Autodesk Fusion 360 part; units mm, degrees
(part 4 of 6)
  spline S7 degree 5 poles (-12.9774, 23.6767) (-12.9776, 23.6654) (-12.9779, 23.6429) (-12.9782, 23.6091) (-12.9786, 23.5641) (-12.9788, 23.5079) (-12.9787, 23.4518) (-12.9784, 23.3958) (-12.9779, 23.3398) (-12.9771, 23.2839) (-12.976, 23.228) (-12.9748, 23.1723) (-12.9732, 23.1166) (-12.9714, 23.061) (-12.9694, 23.0055) (-12.9671, 22.95) (-12.9646, 22.8947) (-12.9618, 22.8394) (-12.9587, 22.7842) (-12.9554, 22.7291) (-12.9519, 22.6741) (-12.948, 22.6192) (-12.9439, 22.5643) (-12.9396, 22.5096) (-12.935, 22.4549) (-12.9301, 22.4004) (-12.9249, 22.3459) (-12.9195, 22.2915) (-12.9138, 22.2373) (-12.9078, 22.1831) (-12.9016, 22.129) (-12.895, 22.0751) (-12.8882, 22.0212) (-12.8811, 21.9675) (-12.8737, 21.9139) (-12.8661, 21.8604) (-12.8581, 21.807) (-12.8498, 21.7537) (-12.8413, 21.7006) (-12.8324, 21.6475) (-12.8233, 21.5946) (-12.8138, 21.5418) (-12.804, 21.4892) (-12.7939, 21.4367) (-12.7835, 21.3843) (-12.7728, 21.3321) (-12.7617, 21.28) (-12.7504, 21.2281) (-12.7387, 21.1763) (-12.7266, 21.1246) (-12.7143, 21.0731) (-12.7015, 21.0218) (-12.6883, 20.9707) (-12.6748, 20.9197) (-12.6609, 20.869) (-12.6466, 20.8184) (-12.632, 20.7679) (-12.617, 20.7177) (-12.6017, 20.6676) (-12.586, 20.6177) (-12.5697, 20.5681) (-12.5529, 20.5187) (-12.5355, 20.4697) (-12.5175, 20.421) (-12.4989, 20.3726) (-12.48, 20.3244) (-12.4607, 20.2763) (-12.4412, 20.2284) (-12.4213, 20.1808) (-12.4005, 20.1336) (-12.3786, 20.0871) (-12.3596, 20.0506) (-12.3444, 20.0238) (-12.3339, 20.0062) (-12.3285, 19.9974) knots -1 -1 -1 -1 -1 -1 -0.98571429 -0.97142857 -0.95714286 -0.94285714 -0.92857143 -0.91428571 -0.9 -0.88571429 -0.87142857 -0.85714286 -0.84285714 -0.82857143 -0.81428571 -0.8 -0.78571429 -0.77142857 -0.75714286 -0.74285714 -0.72857143 -0.71428571 -0.7 -0.68571429 -0.67142857 -0.65714286 -0.64285714 -0.62857143 -0.61428571 -0.6 -0.58571429 -0.57142857 -0.55714286 -0.54285714 -0.52857143 -0.51428571 -0.5 -0.48571429 -0.47142857 -0.45714286 -0.44285714 -0.42857143 -0.41428571 -0.4 -0.38571429 -0.37142857 -0.35714286 -0.34285714 -0.32857143 -0.31428571 -0.3 -0.28571429 -0.27142857 -0.25714286 -0.24285714 -0.22857143 -0.21428571 -0.2 -0.18571429 -0.17142857 -0.15714286 -0.14285714 -0.12857143 -0.11428571 -0.1 -0.08571429 -0.07142857 -0.05714286 -0.04285714 -0.02857143 -0.01428571 0 0 0 0 0 0
  line L7 (-12.3285, 19.9974) -> (-12.0674, 19.5732)
  arc A17 (-12.2216, 18.8913) -> (-12.0674, 19.5732) centre (-12.4932, 19.3111) ccw
  arc A18 (-12.2216, 18.8913) -> (-13.1932, 18.2261) centre (0, 0) ccw
  arc A19 (-13.8847, 18.3289) -> (-13.1932, 18.2261) centre (-13.4864, 18.6311) ccw
  line L8 (-13.8847, 18.3289) -> (-14.1858, 18.7257)
  spline S8 degree 5 poles (-14.1858, 18.7257) (-14.192, 18.7339) (-14.2046, 18.7501) (-14.2242, 18.774) (-14.2513, 18.8048) (-14.2867, 18.8421) (-14.3232, 18.8785) (-14.3604, 18.9144) (-14.398, 18.9499) (-14.4358, 18.9852) (-14.4739, 19.0203) (-14.5124, 19.0551) (-14.5513, 19.0895) (-14.5907, 19.1235) (-14.6306, 19.157) (-14.671, 19.1901) (-14.7118, 19.2228) (-14.753, 19.2552) (-14.7944, 19.2873) (-14.8361, 19.3192) (-14.8781, 19.3508) (-14.9204, 19.3821) (-14.963, 19.4131) (-15.006, 19.4439) (-15.0492, 19.4744) (-15.0927, 19.5045) (-15.1365, 19.5344) (-15.1806, 19.5641) (-15.2249, 19.5935) (-15.2695, 19.6226) (-15.3143, 19.6515) (-15.3593, 19.6801) (-15.4046, 19.7085) (-15.4502, 19.7367) (-15.496, 19.7646) (-15.542, 19.7923) (-15.5882, 19.8197) (-15.6347, 19.8469) (-15.6814, 19.8739) (-15.7283, 19.9006) (-15.7754, 19.9271) (-15.8227, 19.9534) (-15.8702, 19.9794) (-15.918, 20.0052) (-15.9659, 20.0308) (-16.014, 20.0562) (-16.0624, 20.0814) (-16.1109, 20.1063) (-16.1596, 20.131) (-16.2085, 20.1555) (-16.2576, 20.1798) (-16.3069, 20.2039) (-16.3564, 20.2278) (-16.406, 20.2514) (-16.4559, 20.2748) (-16.5059, 20.2981) (-16.5561, 20.3211) (-16.6064, 20.3439) (-16.6569, 20.3665) (-16.7076, 20.3889) (-16.7585, 20.411) (-16.8095, 20.433) (-16.8607, 20.4548) (-16.9121, 20.4763) (-16.9636, 20.4977) (-17.0153, 20.5189) (-17.0671, 20.5398) (-17.1191, 20.5606) (-17.1713, 20.5811) (-17.2236, 20.6014) (-17.276, 20.6216) (-17.3181, 20.6375) (-17.3497, 20.6494) (-17.3709, 20.6573) (-17.3814, 20.6612) knots 0 0 0 0 0 0 0.01428571 0.02857143 0.04285714 0.05714286 0.07142857 0.08571429 0.1 0.11428571 0.12857143 0.14285714 0.15714286 0.17142857 0.18571429 0.2 0.21428571 0.22857143 0.24285714 0.25714286 0.27142857 0.28571429 0.3 0.31428571 0.32857143 0.34285714 0.35714286 0.37142857 0.38571429 0.4 0.41428571 0.42857143 0.44285714 0.45714286 0.47142857 0.48571429 0.5 0.51428571 0.52857143 0.54285714 0.55714286 0.57142857 0.58571429 0.6 0.61428571 0.62857143 0.64285714 0.65714286 0.67142857 0.68571429 0.7 0.71428571 0.72857143 0.74285714 0.75714286 0.77142857 0.78571429 0.8 0.81428571 0.82857143 0.84285714 0.85714286 0.87142857 0.88571429 0.9 0.91428571 0.92857143 0.94285714 0.95714286 0.97142857 0.98571429 1 1 1 1 1 1
  arc A20 (-17.3814, 20.6612) -> (-18.4579, 19.7055) centre (0, 0) ccw
  spline S9 degree 5 poles (-18.4579, 19.7055) (-18.4552, 19.6946) (-18.4499, 19.6727) (-18.4418, 19.6398) (-18.431, 19.5962) (-18.4172, 19.5417) (-18.4032, 19.4874) (-18.389, 19.4331) (-18.3745, 19.3791) (-18.3598, 19.3251) (-18.345, 19.2713) (-18.3298, 19.2176) (-18.3145, 19.1641) (-18.299, 19.1106) (-18.2832, 19.0574) (-18.2672, 19.0042) (-18.251, 18.9512) (-18.2345, 18.8984) (-18.2178, 18.8457) (-18.2009, 18.7931) (-18.1838, 18.7407) (-18.1664, 18.6885) (-18.1488, 18.6364) (-18.131, 18.5844) (-18.1129, 18.5327) (-18.0946, 18.481) (-18.0761, 18.4296) (-18.0573, 18.3782) (-18.0383, 18.3271) (-18.019, 18.2761) (-17.9995, 18.2253) (-17.9798, 18.1747) (-17.9598, 18.1242) (-17.9395, 18.074) (-17.919, 18.0239) (-17.8983, 17.9739) (-17.8773, 17.9242) (-17.8561, 17.8746) (-17.8346, 17.8253) (-17.8128, 17.7761) (-17.7908, 17.7272) (-17.7685, 17.6784) (-17.7459, 17.6298) (-17.7231, 17.5815) (-17.7, 17.5334) (-17.6766, 17.4854) (-17.6529, 17.4377) (-17.629, 17.3902) (-17.6048, 17.343) (-17.5803, 17.2959) (-17.5555, 17.2492) (-17.5304, 17.2026) (-17.5049, 17.1564) (-17.4791, 17.1104) (-17.453, 17.0647) (-17.4266, 17.0192) (-17.3999, 16.974) (-17.3729, 16.9291) (-17.3456, 16.8844) (-17.318, 16.84) (-17.2899, 16.7959) (-17.2614, 16.7523) (-17.2323, 16.7092) (-17.2027, 16.6665) (-17.1727, 16.6242) (-17.1424, 16.5822) (-17.1118, 16.5405) (-17.081, 16.4989) (-17.0498, 16.4577) (-17.018, 16.4172) (-16.9851, 16.3776) (-16.9577, 16.347) (-16.9363, 16.3248) (-16.9217, 16.3104) (-16.9143, 16.3032) knots -1 -1 -1 -1 -1 -1 -0.98571429 -0.97142857 -0.95714286 -0.94285714 -0.92857143 -0.91428571 -0.9 -0.88571429 -0.87142857 -0.85714286 -0.84285714 -0.82857143 -0.81428571 -0.8 -0.78571429 -0.77142857 -0.75714286 -0.74285714 -0.72857143 -0.71428571 -0.7 -0.68571429 -0.67142857 -0.65714286 -0.64285714 -0.62857143 -0.61428571 -0.6 -0.58571429 -0.57142857 -0.55714286 -0.54285714 -0.52857143 -0.51428571 -0.5 -0.48571429 -0.47142857 -0.45714286 -0.44285714 -0.42857143 -0.41428571 -0.4 -0.38571429 -0.37142857 -0.35714286 -0.34285714 -0.32857143 -0.31428571 -0.3 -0.28571429 -0.27142857 -0.25714286 -0.24285714 -0.22857143 -0.21428571 -0.2 -0.18571429 -0.17142857 -0.15714286 -0.14285714 -0.12857143 -0.11428571 -0.1 -0.08571429 -0.07142857 -0.05714286 -0.04285714 -0.02857143 -0.01428571 0 0 0 0 0 0
  line L9 (-16.9143, 16.3032) -> (-16.5559, 15.9572)
  arc A21 (-16.5357, 15.2584) -> (-16.5559, 15.9572) centre (-16.9032, 15.5975) ccw
  arc A22 (-16.5357, 15.2584) -> (-17.3113, 14.3724) centre (0, 0) ccw
  arc A23 (-18.0067, 14.3) -> (-17.3113, 14.3724) centre (-17.696, 14.6918) ccw
  line L10 (-18.0067, 14.3) -> (-18.397, 14.6095)
  spline S10 degree 5 poles (-18.397, 14.6095) (-18.4051, 14.6159) (-18.4213, 14.6285) (-18.4462, 14.6467) (-18.4801, 14.6699) (-18.5237, 14.6972) (-18.5681, 14.7234) (-18.6131, 14.7488) (-18.6583, 14.7739) (-18.7037, 14.7987) (-18.7494, 14.8232) (-18.7953, 14.8474) (-18.8415, 14.871) (-18.8881, 14.8941) (-18.9351, 14.9166) (-18.9824, 14.9386) (-19.0301, 14.9602) (-19.078, 14.9813) (-19.1262, 15.0021) (-19.1745, 15.0226) (-19.2231, 15.0428) (-19.2718, 15.0626) (-19.3208, 15.0821) (-19.37, 15.1012) (-19.4195, 15.12) (-19.4691, 15.1384) (-19.519, 15.1564) (-19.569, 15.1742) (-19.6193, 15.1916) (-19.6697, 15.2088) (-19.7203, 15.2256) (-19.771, 15.2421) (-19.822, 15.2584) (-19.8731, 15.2743) (-19.9244, 15.29) (-19.9758, 15.3053) (-20.0274, 15.3204) (-20.0792, 15.3352) (-20.1311, 15.3497) (-20.1832, 15.3639) (-20.2354, 15.3779) (-20.2878, 15.3915) (-20.3403, 15.405) (-20.393, 15.4181) (-20.4458, 15.431) (-20.4987, 15.4436) (-20.5518, 15.4559) (-20.605, 15.468) (-20.6583, 15.4798) (-20.7118, 15.4914) (-20.7654, 15.5027) (-20.8191, 15.5138) (-20.873, 15.5246) (-20.9269, 15.5352) (-20.981, 15.5455) (-21.0352, 15.5555) (-21.0896, 15.5653) (-21.144, 15.5749) (-21.1986, 15.5842) (-21.2532, 15.5933) (-21.308, 15.6021) (-21.3629, 15.6107) (-21.4179, 15.6191) (-21.473, 15.6272) (-21.5282, 15.6351) (-21.5836, 15.6427) (-21.639, 15.6501) (-21.6945, 15.6573) (-21.7501, 15.6642) (-21.8058, 15.6709) (-21.8616, 15.6774) (-21.9064, 15.6823) (-21.94, 15.686) (-21.9624, 15.6884) (-21.9736, 15.6895) knots 0 0 0 0 0 0 0.01428571 0.02857143 0.04285714 0.05714286 0.07142857 0.08571429 0.1 0.11428571 0.12857143 0.14285714 0.15714286 0.17142857 0.18571429 0.2 0.21428571 0.22857143 0.24285714 0.25714286 0.27142857 0.28571429 0.3 0.31428571 0.32857143 0.34285714 0.35714286 0.37142857 0.38571429 0.4 0.41428571 0.42857143 0.44285714 0.45714286 0.47142857 0.48571429 0.5 0.51428571 0.52857143 0.54285714 0.55714286 0.57142857 0.58571429 0.6 0.61428571 0.62857143 0.64285714 0.65714286 0.67142857 0.68571429 0.7 0.71428571 0.72857143 0.74285714 0.75714286 0.77142857 0.78571429 0.8 0.81428571 0.82857143 0.84285714 0.85714286 0.87142857 0.88571429 0.9 0.91428571 0.92857143 0.94285714 0.95714286 0.97142857 0.98571429 1 1 1 1 1 1
  arc A24 (-21.9736, 15.6895) -> (-22.7785, 14.4962) centre (0, 0) ccw
  spline S11 degree 5 poles (-22.7785, 14.4962) (-22.7732, 14.4862) (-22.7626, 14.4663) (-22.7467, 14.4365) (-22.7253, 14.3969) (-22.6984, 14.3476) (-22.6713, 14.2984) (-22.6441, 14.2495) (-22.6166, 14.2007) (-22.589, 14.1521) (-22.5612, 14.1036) (-22.5332, 14.0554) (-22.505, 14.0073) (-22.4767, 13.9595) (-22.4482, 13.9118) (-22.4194, 13.8643) (-22.3906, 13.817) (-22.3615, 13.7699) (-22.3322, 13.723) (-22.3028, 13.6763) (-22.2731, 13.6298) (-22.2433, 13.5836) (-22.2133, 13.5375) (-22.1831, 13.4916) (-22.1527, 13.4459) (-22.1222, 13.4005) (-22.0914, 13.3552) (-22.0605, 13.3102) (-22.0293, 13.2654) (-21.998, 13.2208) (-21.9665, 13.1764) (-21.9348, 13.1323) (-21.9028, 13.0884) (-21.8707, 13.0447) (-21.8384, 13.0013) (-21.8059, 12.9581) (-21.7732, 12.9152) (-21.7403, 12.8725) (-21.7072, 12.83) (-21.6739, 12.7878) (-21.6404, 12.7458) (-21.6067, 12.7041) (-21.5728, 12.6627) (-21.5386, 12.6216) (-21.5043, 12.5807) (-21.4697, 12.5401) (-21.4349, 12.4998) (-21.3999, 12.4597) (-21.3647, 12.42) (-21.3293, 12.3805) (-21.2936, 12.3414) (-21.2577, 12.3026) (-21.2216, 12.2641) (-21.1852, 12.226) (-21.1485, 12.1882) (-21.1116, 12.1507) (-21.0745, 12.1136) (-21.0372, 12.0767) (-20.9996, 12.0402) (-20.9618, 12.0041) (-20.9237, 11.9684) (-20.8852, 11.9333) (-20.8463, 11.8987) (-20.8071, 11.8647) (-20.7675, 11.8312) (-20.7276, 11.7981) (-20.6876, 11.7653) (-20.6475, 11.7327) (-20.607, 11.7006) (-20.5661, 11.6692) (-20.5245, 11.639) (-20.4903, 11.6162) (-20.4641, 11.6) (-20.4463, 11.5897) (-20.4374, 11.5846) knots -1 -1 -1 -1 -1 -1 -0.98571429 -0.97142857 -0.95714286 -0.94285714 -0.92857143 -0.91428571 -0.9 -0.88571429 -0.87142857 -0.85714286 -0.84285714 -0.82857143 -0.81428571 -0.8 -0.78571429 -0.77142857 -0.75714286 -0.74285714 -0.72857143 -0.71428571 -0.7 -0.68571429 -0.67142857 -0.65714286 -0.64285714 -0.62857143 -0.61428571 -0.6 -0.58571429 -0.57142857 -0.55714286 -0.54285714 -0.52857143 -0.51428571 -0.5 -0.48571429 -0.47142857 -0.45714286 -0.44285714 -0.42857143 -0.41428571 -0.4 -0.38571429 -0.37142857 -0.35714286 -0.34285714 -0.32857143 -0.31428571 -0.3 -0.28571429 -0.27142857 -0.25714286 -0.24285714 -0.22857143 -0.21428571 -0.2 -0.18571429 -0.17142857 -0.15714286 -0.14285714 -0.12857143 -0.11428571 -0.1 -0.08571429 -0.07142857 -0.05714286 -0.04285714 -0.02857143 -0.01428571 0 0 0 0 0 0
  line L11 (-20.4374, 11.5846) -> (-20.0042, 11.3386)
  arc A25 (-19.8108, 10.6668) -> (-20.0042, 11.3386) centre (-20.2511, 10.9038) ccw
  arc A26 (-19.8108, 10.6668) -> (-20.3418, 9.6158) centre (0, 0) ccw
  arc A27 (-20.9972, 9.3727) -> (-20.3418, 9.6158) centre (-20.7938, 9.8294) ccw
  line L12 (-20.9972, 9.3727) -> (-21.4523, 9.5754)
  spline S12 degree 5 poles (-21.4523, 9.5754) (-21.4617, 9.5796) (-21.4806, 9.5877) (-21.5092, 9.5992) (-21.5478, 9.6132) (-21.5968, 9.6288) (-21.6463, 9.6431) (-21.6962, 9.6566) (-21.7462, 9.6696) (-21.7964, 9.6823) (-21.8467, 9.6947) (-21.8972, 9.7067) (-21.9478, 9.7181) (-21.9987, 9.7289) (-22.0498, 9.7391) (-22.1012, 9.7486) (-22.1527, 9.7576) (-22.2044, 9.7661) (-22.2562, 9.7743) (-22.3081, 9.7821) (-22.3601, 9.7896) (-22.4123, 9.7967) (-22.4646, 9.8034) (-22.517, 9.8096) (-22.5695, 9.8155) (-22.6222, 9.821) (-22.675, 9.8261) (-22.7279, 9.8308) (-22.7809, 9.8352) (-22.834, 9.8393) (-22.8872, 9.843) (-22.9405, 9.8464) (-22.9938, 9.8495) (-23.0473, 9.8522) (-23.1009, 9.8546) (-23.1545, 9.8567) (-23.2083, 9.8585) (-23.2621, 9.8599) (-23.316, 9.861) (-23.37, 9.8619) (-23.424, 9.8624) (-23.4781, 9.8626) (-23.5323, 9.8626) (-23.5866, 9.8622) (-23.641, 9.8615) (-23.6954, 9.8606) (-23.7498, 9.8593) (-23.8044, 9.8578) (-23.859, 9.856) (-23.9137, 9.8539) (-23.9684, 9.8515) (-24.0232, 9.8489) (-24.078, 9.846) (-24.1329, 9.8428) (-24.1879, 9.8393) (-24.2429, 9.8356) (-24.2979, 9.8316) (-24.3531, 9.8273) (-24.4082, 9.8227) (-24.4634, 9.8179) (-24.5187, 9.8129) (-24.574, 9.8075) (-24.6293, 9.8019) (-24.6847, 9.7961) (-24.7402, 9.79) (-24.7956, 9.7836) (-24.8512, 9.777) (-24.9067, 9.7702) (-24.9623, 9.763) (-25.0179, 9.7557) (-25.0736, 9.7481) (-25.1182, 9.7418) (-25.1516, 9.7369) (-25.1739, 9.7337) (-25.1851, 9.732) knots 0 0 0 0 0 0 0.01428571 0.02857143 0.04285714 0.05714286 0.07142857 0.08571429 0.1 0.11428571 0.12857143 0.14285714 0.15714286 0.17142857 0.18571429 0.2 0.21428571 0.22857143 0.24285714 0.25714286 0.27142857 0.28571429 0.3 0.31428571 0.32857143 0.34285714 0.35714286 0.37142857 0.38571429 0.4 0.41428571 0.42857143 0.44285714 0.45714286 0.47142857 0.48571429 0.5 0.51428571 0.52857143 0.54285714 0.55714286 0.57142857 0.58571429 0.6 0.61428571 0.62857143 0.64285714 0.65714286 0.67142857 0.68571429 0.7 0.71428571 0.72857143 0.74285714 0.75714286 0.77142857 0.78571429 0.8 0.81428571 0.82857143 0.84285714 0.85714286 0.87142857 0.88571429 0.9 0.91428571 0.92857143 0.94285714 0.95714286 0.97142857 0.98571429 1 1 1 1 1 1
  arc A28 (-25.1851, 9.732) -> (-25.6679, 8.3759) centre (0, 0) ccw
  spline S13 degree 5 poles (-25.6679, 8.3759) (-25.6603, 8.3676) (-25.6451, 8.351) (-25.6223, 8.3261) (-25.5917, 8.2931) (-25.5534, 8.252) (-25.5149, 8.2111) (-25.4763, 8.1704) (-25.4376, 8.13) (-25.3988, 8.0898) (-25.3598, 8.0498) (-25.3207, 8.01) (-25.2815, 7.9705) (-25.2421, 7.9312) (-25.2026, 7.8921) (-25.163, 7.8533) (-25.1233, 7.8146) (-25.0834, 7.7763) (-25.0434, 7.7381) (-25.0033, 7.7002) (-24.963, 7.6625) (-24.9226, 7.6251) (-24.8821, 7.5879) (-24.8414, 7.551) (-24.8006, 7.5143) (-24.7597, 7.4779) (-24.7187, 7.4417) (-24.6775, 7.4058) (-24.6362, 7.3702) (-24.5948, 7.3348) (-24.5532, 7.2996) (-24.5115, 7.2648) (-24.4697, 7.2302) (-24.4277, 7.1959) (-24.3856, 7.1619) (-24.3434, 7.1281) (-24.3011, 7.0946) (-24.2586, 7.0614) (-24.216, 7.0286) (-24.1732, 6.9959) (-24.1303, 6.9636) (-24.0873, 6.9317) (-24.0441, 6.9) (-24.0008, 6.8686) (-23.9574, 6.8376) (-23.9138, 6.8068) (-23.8701, 6.7764) (-23.8262, 6.7464) (-23.7822, 6.7166) (-23.7381, 6.6872) (-23.6938, 6.6581) (-23.6494, 6.6295) (-23.6048, 6.6012) (-23.5601, 6.5733) (-23.5152, 6.5459) (-23.4701, 6.5187) (-23.4249, 6.492) (-23.3796, 6.4656) (-23.3342, 6.4396) (-23.2886, 6.414) (-23.2428, 6.3889) (-23.1967, 6.3645) (-23.1505, 6.3406) (-23.104, 6.3175) (-23.0573, 6.2949) (-23.0105, 6.2727) (-22.9636, 6.2508) (-22.9166, 6.2293) (-22.8694, 6.2082) (-22.822, 6.188) (-22.7742, 6.1691) (-22.7354, 6.1556) (-22.706, 6.1464) (-22.6862, 6.1408) (-22.6763, 6.1381) knots -1 -1 -1 -1 -1 -1 -0.98571429 -0.97142857 -0.95714286 -0.94285714 -0.92857143 -0.91428571 -0.9 -0.88571429 -0.87142857 -0.85714286 -0.84285714 -0.82857143 -0.81428571 -0.8 -0.78571429 -0.77142857 -0.75714286 -0.74285714 -0.72857143 -0.71428571 -0.7 -0.68571429 -0.67142857 -0.65714286 -0.64285714 -0.62857143 -0.61428571 -0.6 -0.58571429 -0.57142857 -0.55714286 -0.54285714 -0.52857143 -0.51428571 -0.5 -0.48571429 -0.47142857 -0.45714286 -0.44285714 -0.42857143 -0.41428571 -0.4 -0.38571429 -0.37142857 -0.35714286 -0.34285714 -0.32857143 -0.31428571 -0.3 -0.28571429 -0.27142857 -0.25714286 -0.24285714 -0.22857143 -0.21428571 -0.2 -0.18571429 -0.17142857 -0.15714286 -0.14285714 -0.12857143 -0.11428571 -0.1 -0.08571429 -0.07142857 -0.05714286 -0.04285714 -0.02857143 -0.01428571 0 0 0 0 0 0
  line L13 (-22.6763, 6.1381) -> (-22.1955, 6.0076)
  arc A29 (-21.8412, 5.4049) -> (-22.1955, 6.0076) centre (-22.3265, 5.525) ccw
  arc A30 (-21.8412, 5.4049) -> (-22.094, 4.2549) centre (0, 0) ccw
  arc A31 (-22.6685, 3.8564) -> (-22.094, 4.2549) centre (-22.585, 4.3494) ccw
  line L14 (-22.6685, 3.8564) -> (-23.1596, 3.9396)
  spline S14 degree 5 poles (-23.1596, 3.9396) (-23.1698, 3.9413) (-23.1901, 3.9445) (-23.2206, 3.9485) (-23.2615, 3.9525) (-23.3129, 3.9554) (-23.3644, 3.9569) (-23.4161, 3.9576) (-23.4678, 3.9578) (-23.5195, 3.9576) (-23.5713, 3.9571) (-23.6232, 3.9562) (-23.6751, 3.9546) (-23.7271, 3.9524) (-23.7791, 3.9495) (-23.8312, 3.946) (-23.8833, 3.9419) (-23.9355, 3.9373) (-23.9877, 3.9324) (-24.04, 3.927) (-24.0922, 3.9213) (-24.1445, 3.9152) (-24.1968, 3.9087) (-24.2491, 3.9017) (-24.3015, 3.8943) (-24.3539, 3.8865) (-24.4063, 3.8783) (-24.4587, 3.8698) (-24.5111, 3.8609) (-24.5635, 3.8516) (-24.616, 3.842) (-24.6685, 3.832) (-24.7209, 3.8217) (-24.7734, 3.8111) (-24.8259, 3.8001) (-24.8783, 3.7887) (-24.9308, 3.7771) (-24.9833, 3.7651) (-25.0358, 3.7528) (-25.0883, 3.7402) (-25.1408, 3.7272) (-25.1933, 3.714) (-25.2458, 3.7004) (-25.2982, 3.6866) (-25.3507, 3.6724) (-25.4032, 3.658) (-25.4556, 3.6432) (-25.5081, 3.6282) (-25.5605, 3.6129) (-25.6129, 3.5972) (-25.6654, 3.5813) (-25.7178, 3.5652) (-25.7702, 3.5487) (-25.8225, 3.5319) (-25.8749, 3.5149) (-25.9273, 3.4976) (-25.9796, 3.48) (-26.0319, 3.4622) (-26.0842, 3.4441) (-26.1365, 3.4257) (-26.1887, 3.407) (-26.241, 3.3881) (-26.2932, 3.3689) (-26.3454, 3.3495) (-26.3976, 3.3298) (-26.4497, 3.3098) (-26.5019, 3.2896) (-26.554, 3.2692) (-26.606, 3.2484) (-26.6581, 3.2275) (-26.7101, 3.2062) (-26.7517, 3.1891) (-26.7829, 3.1761) (-26.8037, 3.1674) (-26.8141, 3.163) knots 0 0 0 0 0 0 0.01428571 0.02857143 0.04285714 0.05714286 0.07142857 0.08571429 0.1 0.11428571 0.12857143 0.14285714 0.15714286 0.17142857 0.18571429 0.2 0.21428571 0.22857143 0.24285714 0.25714286 0.27142857 0.28571429 0.3 0.31428571 0.32857143 0.34285714 0.35714286 0.37142857 0.38571429 0.4 0.41428571 0.42857143 0.44285714 0.45714286 0.47142857 0.48571429 0.5 0.51428571 0.52857143 0.54285714 0.55714286 0.57142857 0.58571429 0.6 0.61428571 0.62857143 0.64285714 0.65714286 0.67142857 0.68571429 0.7 0.71428571 0.72857143 0.74285714 0.75714286 0.77142857 0.78571429 0.8 0.81428571 0.82857143 0.84285714 0.85714286 0.87142857 0.88571429 0.9 0.91428571 0.92857143 0.94285714 0.95714286 0.97142857 0.98571429 1 1 1 1 1 1
  arc A32 (-26.8141, 3.163) -> (-26.9446, 1.7294) centre (0, 0) ccw
  spline S15 degree 5 poles (-26.9446, 1.7294) (-26.9351, 1.7233) (-26.9163, 1.7109) (-26.8879, 1.6925) (-26.8501, 1.6681) (-26.8028, 1.6379) (-26.7554, 1.6078) (-26.7079, 1.578) (-26.6603, 1.5485) (-26.6127, 1.5192) (-26.565, 1.4902) (-26.5172, 1.4614) (-26.4694, 1.4328) (-26.4215, 1.4046) (-26.3735, 1.3765) (-26.3255, 1.3487) (-26.2774, 1.3212) (-26.2292, 1.294) (-26.181, 1.267) (-26.1327, 1.2402) (-26.0843, 1.2138) (-26.0359, 1.1876) (-25.9874, 1.1616) (-25.9388, 1.136) (-25.8902, 1.1106) (-25.8415, 1.0855) (-25.7928, 1.0606) (-25.744, 1.0361) (-25.6951, 1.0118) (-25.6462, 0.9879) (-25.5972, 0.9642) (-25.5481, 0.9408) (-25.499, 0.9177) (-25.4498, 0.8949) (-25.4006, 0.8724) (-25.3513, 0.8502) (-25.302, 0.8283) (-25.2526, 0.8067) (-25.2031, 0.7855) (-25.1536, 0.7645) (-25.104, 0.7439) (-25.0544, 0.7236) (-25.0047, 0.7037) (-24.9549, 0.6841) (-24.9051, 0.6648) (-24.8553, 0.6459) (-24.8054, 0.6273) (-24.7554, 0.6091) (-24.7054, 0.5912) (-24.6554, 0.5737) (-24.6053, 0.5565) (-24.5551, 0.5398) (-24.5049, 0.5235) (-24.4546, 0.5077) (-24.4043, 0.4922) (-24.3539, 0.4772) (-24.3035, 0.4625) (-24.253, 0.4482) (-24.2025, 0.4343) (-24.152, 0.4208) (-24.1014, 0.408) (-24.0507, 0.3957) (-24, 0.3842) (-23.9492, 0.3733) (-23.8984, 0.363) (-23.8476, 0.3531) (-23.7967, 0.3436) (-23.7458, 0.3345) (-23.6949, 0.3258) (-23.6439, 0.318) (-23.5929, 0.3116) (-23.5519, 0.3081) (-23.5212, 0.3066) (-23.5006, 0.306) (-23.4903, 0.3059) knots -1 -1 -1 -1 -1 -1 -0.98571429 -0.97142857 -0.95714286 -0.94285714 -0.92857143 -0.91428571 -0.9 -0.88571429 -0.87142857 -0.85714286 -0.84285714 -0.82857143 -0.81428571 -0.8 -0.78571429 -0.77142857 -0.75714286 -0.74285714 -0.72857143 -0.71428571 -0.7 -0.68571429 -0.67142857 -0.65714286 -0.64285714 -0.62857143 -0.61428571 -0.6 -0.58571429 -0.57142857 -0.55714286 -0.54285714 -0.52857143 -0.51428571 -0.5 -0.48571429 -0.47142857 -0.45714286 -0.44285714 -0.42857143 -0.41428571 -0.4 -0.38571429 -0.37142857 -0.35714286 -0.34285714 -0.32857143 -0.31428571 -0.3 -0.28571429 -0.27142857 -0.25714286 -0.24285714 -0.22857143 -0.21428571 -0.2 -0.18571429 -0.17142857 -0.15714286 -0.14285714 -0.12857143 -0.11428571 -0.1 -0.08571429 -0.07142857 -0.05714286 -0.04285714 -0.02857143 -0.01428571 0 0 0 0 0 0
  line L15 (-23.4903, 0.3059) -> (-22.9922, 0.299)
  arc A33 (-22.4991, -0.1966) -> (-22.9922, 0.299) centre (-22.9991, -0.2009) ccw
  arc A34 (-22.4991, -0.1966) -> (-22.458, -1.3734) centre (0, 0) ccw
  arc A35 (-22.9154, -1.9021) -> (-22.458, -1.3734) centre (-22.9571, -1.4039) ccw
  line L16 (-22.9154, -1.9021) -> (-23.4118, -1.9437)
  spline S16 degree 5 poles (-23.4118, -1.9437) (-23.422, -1.9446) (-23.4425, -1.9466) (-23.4731, -1.9503) (-23.5137, -1.9566) (-23.5641, -1.9665) (-23.6144, -1.9779) (-23.6646, -1.9901) (-23.7147, -2.0028) (-23.7648, -2.0158) (-23.8149, -2.0292) (-23.8649, -2.043) (-23.9148, -2.0574) (-23.9646, -2.0724) (-24.0142, -2.0882) (-24.0638, -2.1046) (-24.1133, -2.1215) (-24.1627, -2.1389) (-24.212, -2.1567) (-24.2613, -2.1748) (-24.3105, -2.1934) (-24.3596, -2.2123) (-24.4087, -2.2316) (-24.4576, -2.2514) (-24.5065, -2.2716) (-24.5553, -2.2921) (-24.604, -2.3131) (-24.6526, -2.3344) (-24.7012, -2.3561) (-24.7497, -2.3781) (-24.7981, -2.4005) (-24.8464, -2.4232) (-24.8947, -2.4462) (-24.9429, -2.4696) (-24.991, -2.4933) (-25.039, -2.5173) (-25.0869, -2.5416) (-25.1348, -2.5663) (-25.1825, -2.5913) (-25.2302, -2.6165) (-25.2779, -2.6421) (-25.3254, -2.668) (-25.3729, -2.6942) (-25.4203, -2.7206) (-25.4676, -2.7474) (-25.5148, -2.7744) (-25.5619, -2.8018) (-25.609, -2.8294) (-25.656, -2.8573) (-25.7029, -2.8854) (-25.7497, -2.9139) (-25.7964, -2.9426) (-25.8431, -2.9716) (-25.8896, -3.0008) (-25.9361, -3.0304) (-25.9825, -3.0601) (-26.0288, -3.0902) (-26.0751, -3.1205) (-26.1212, -3.151) (-26.1673, -3.1818) (-26.2133, -3.2129) (-26.2592, -3.2442) (-26.305, -3.2758) (-26.3507, -3.3076) (-26.3963, -3.3396) (-26.4419, -3.3719) (-26.4874, -3.4045) (-26.5327, -3.4373) (-26.578, -3.4703) (-26.6232, -3.5035) (-26.6683, -3.537) (-26.7044, -3.564) (-26.7313, -3.5844) (-26.7493, -3.598) (-26.7583, -3.6048) knots 0 0 0 0 0 0 0.01428571 0.02857143 0.04285714 0.05714286 0.07142857 0.08571429 0.1 0.11428571 0.12857143 0.14285714 0.15714286 0.17142857 0.18571429 0.2 0.21428571 0.22857143 0.24285714 0.25714286 0.27142857 0.28571429 0.3 0.31428571 0.32857143 0.34285714 0.35714286 0.37142857 0.38571429 0.4 0.41428571 0.42857143 0.44285714 0.45714286 0.47142857 0.48571429 0.5 0.51428571 0.52857143 0.54285714 0.55714286 0.57142857 0.58571429 0.6 0.61428571 0.62857143 0.64285714 0.65714286 0.67142857 0.68571429 0.7 0.71428571 0.72857143 0.74285714 0.75714286 0.77142857 0.78571429 0.8 0.81428571 0.82857143 0.84285714 0.85714286 0.87142857 0.88571429 0.9 0.91428571 0.92857143 0.94285714 0.95714286 0.97142857 0.98571429 1 1 1 1 1 1
  arc A36 (-26.7583, -3.6048) -> (-26.5281, -5.0257) centre (0, 0) ccw
  spline S17 degree 5 poles (-26.5281, -5.0257) (-26.5175, -5.0294) (-26.4961, -5.0366) (-26.4641, -5.0474) (-26.4214, -5.0616) (-26.368, -5.0792) (-26.3146, -5.0965) (-26.2612, -5.1135) (-26.2078, -5.1303) (-26.1544, -5.1468) (-26.101, -5.1631) (-26.0476, -5.1791) (-25.9942, -5.1948) (-25.9407, -5.2103) (-25.8873, -5.2256) (-25.8339, -5.2405) (-25.7804, -5.2552) (-25.727, -5.2696) (-25.6735, -5.2838) (-25.6201, -5.2977) (-25.5667, -5.3113) (-25.5133, -5.3246) (-25.4598, -5.3377) (-25.4064, -5.3504) (-25.353, -5.3629) (-25.2996, -5.3752) (-25.2462, -5.3871) (-25.1928, -5.3987) (-25.1395, -5.4101) (-25.0861, -5.4211) (-25.0328, -5.4319) (-24.9794, -5.4423) (-24.9261, -5.4525) (-24.8728, -5.4623) (-24.8195, -5.4719) (-24.7663, -5.4811) (-24.713, -5.4901) (-24.6598, -5.4987) (-24.6066, -5.507) (-24.5535, -5.5149) (-24.5003, -5.5226) (-24.4472, -5.5299) (-24.3941, -5.5368) (-24.3411, -5.5435) (-24.288, -5.5497) (-24.235, -5.5557) (-24.1821, -5.5613) (-24.1292, -5.5665) (-24.0763, -5.5714) (-24.0234, -5.5759) (-23.9706, -5.58) (-23.9179, -5.5837) (-23.8652, -5.587) (-23.8126, -5.5899) (-23.76, -5.5923) (-23.7075, -5.5944) (-23.655, -5.5961) (-23.6026, -5.5974) (-23.5502, -5.5983) (-23.4979, -5.5987) (-23.4457, -5.5986) (-23.3936, -5.5979) (-23.3416, -5.5965) (-23.2897, -5.5944) (-23.2379, -5.5917) (-23.1862, -5.5886) (-23.1345, -5.5851) (-23.0829, -5.5814) (-23.0315, -5.5771) (-22.9802, -5.572) (-22.9292, -5.5655) (-22.8886, -5.5587) (-22.8584, -5.5525) (-22.8384, -5.548) (-22.8284, -5.5455) knots -1 -1 -1 -1 -1 -1 -0.98571429 -0.97142857 -0.95714286 -0.94285714 -0.92857143 -0.91428571 -0.9 -0.88571429 -0.87142857 -0.85714286 -0.84285714 -0.82857143 -0.81428571 -0.8 -0.78571429 -0.77142857 -0.75714286 -0.74285714 -0.72857143 -0.71428571 -0.7 -0.68571429 -0.67142857 -0.65714286 -0.64285714 -0.62857143 -0.61428571 -0.6 -0.58571429 -0.57142857 -0.55714286 -0.54285714 -0.52857143 -0.51428571 -0.5 -0.48571429 -0.47142857 -0.45714286 -0.44285714 -0.42857143 -0.41428571 -0.4 -0.38571429 -0.37142857 -0.35714286 -0.34285714 -0.32857143 -0.31428571 -0.3 -0.28571429 -0.27142857 -0.25714286 -0.24285714 -0.22857143 -0.21428571 -0.2 -0.18571429 -0.17142857 -0.15714286 -0.14285714 -0.12857143 -0.11428571 -0.1 -0.08571429 -0.07142857 -0.05714286 -0.04285714 -0.02857143 -0.01428571 0 0 0 0 0 0
  line L17 (-22.8284, -5.5455) -> (-22.3442, -5.4283)
  arc A37 (-21.7434, -5.7857) -> (-22.3442, -5.4283) centre (-22.2266, -5.9143) ccw
  arc A38 (-21.7434, -5.7857) -> (-21.5846, -6.3527) centre (0, 0) ccw
  line L18 (-21.5846, -6.3527) -> (-32.7755, -11.2419)
  arc A39 (-38.1149, -11.9886) -> (-32.7755, -11.2419) centre (-36.779, -2.0783) ccw
  arc A40 (-38.1149, -11.9886) -> (-34.6932, -19.8205) centre (-38.7828, -16.9438) ccw
  arc A41 (-30.5175, -16.4102) -> (-34.6932, -19.8205) centre (-26.514, -25.5738) ccw
  line L19 (-30.5175, -16.4102) -> (-19.3266, -11.521)
  arc A42 (-19.3266, -11.521) -> (-19.0185, -12.0227) centre (0, 0) ccw
  arc A43 (-19.1645, -12.7064) -> (-19.0185, -12.0227) centre (-19.4411, -12.2899) ccw
  line L20 (-19.1645, -12.7064) -> (-19.5795, -12.982)
  spline S18 degree 5 poles (-19.5795, -12.982) (-19.588, -12.9877) (-19.605, -12.9993) (-19.6301, -13.0173) (-19.6626, -13.0424) (-19.702, -13.0754) (-19.7406, -13.1096) (-19.7787, -13.1444) (-19.8165, -13.1797) (-19.8542, -13.2153) (-19.8916, -13.2511) (-19.9287, -13.2873) (-19.9655, -13.3239) (-20.0019, -13.3611) (-20.0378, -13.3988) (-20.0734, -13.4371) (-20.1086, -13.4758) (-20.1435, -13.5148) (-20.1782, -13.5542) (-20.2126, -13.5938) (-20.2468, -13.6337) (-20.2807, -13.674) (-20.3144, -13.7146) (-20.3478, -13.7555) (-20.3809, -13.7967) (-20.4137, -13.8382) (-20.4463, -13.8801) (-20.4787, -13.9222) (-20.5108, -13.9646) (-20.5426, -14.0072) (-20.5743, -14.0501) (-20.6057, -14.0933) (-20.6369, -14.1367) (-20.6679, -14.1804) (-20.6986, -14.2243) (-20.7291, -14.2685) (-20.7594, -14.313) (-20.7894, -14.3576) (-20.8193, -14.4025) (-20.8489, -14.4477) (-20.8783, -14.493) (-20.9075, -14.5386) (-20.9365, -14.5844) (-20.9653, -14.6304) (-20.9938, -14.6767) (-21.0222, -14.7231) (-21.0503, -14.7698) (-21.0783, -14.8166) (-21.106, -14.8637) (-21.1335, -14.911) (-21.1608, -14.9585) (-21.188, -15.0061) (-21.2149, -15.054) (-21.2416, -15.1021) (-21.2681, -15.1503) (-21.2944, -15.1988) (-21.3205, -15.2474) (-21.3465, -15.2962) (-21.3722, -15.3453) (-21.3977, -15.3944) (-21.423, -15.4438) (-21.4482, -15.4934) (-21.4731, -15.5431) (-21.4979, -15.593) (-21.5224, -15.6431) (-21.5468, -15.6933) (-21.5709, -15.7437) (-21.5949, -15.7943) (-21.6187, -15.8451) (-21.6423, -15.896) (-21.6657, -15.9471) (-21.6842, -15.9881) (-21.6981, -16.0189) (-21.7073, -16.0395) (-21.7118, -16.0498) knots 0 0 0 0 0 0 0.01428571 0.02857143 0.04285714 0.05714286 0.07142857 0.08571429 0.1 0.11428571 0.12857143 0.14285714 0.15714286 0.17142857 0.18571429 0.2 0.21428571 0.22857143 0.24285714 0.25714286 0.27142857 0.28571429 0.3 0.31428571 0.32857143 0.34285714 0.35714286 0.37142857 0.38571429 0.4 0.41428571 0.42857143 0.44285714 0.45714286 0.47142857 0.48571429 0.5 0.51428571 0.52857143 0.54285714 0.55714286 0.57142857 0.58571429 0.6 0.61428571 0.62857143 0.64285714 0.65714286 0.67142857 0.68571429 0.7 0.71428571 0.72857143 0.74285714 0.75714286 0.77142857 0.78571429 0.8 0.81428571 0.82857143 0.84285714 0.85714286 0.87142857 0.88571429 0.9 0.91428571 0.92857143 0.94285714 0.95714286 0.97142857 0.98571429 1 1 1 1 1 1
  arc A44 (-21.7118, -16.0498) -> (-20.8256, -17.1841) centre (0, 0) ccw
  spline S19 degree 5 poles (-20.8256, -17.1841) (-20.8145, -17.1822) (-20.7923, -17.1782) (-20.7591, -17.1722) (-20.7148, -17.1642) (-20.6596, -17.1538) (-20.6044, -17.1432) (-20.5494, -17.1324) (-20.4946, -17.1214) (-20.4398, -17.1102) (-20.3851, -17.0987) (-20.3306, -17.087) (-20.2762, -17.0751) (-20.2219, -17.0629) (-20.1678, -17.0505) (-20.1137, -17.0379) (-20.0598, -17.025) (-20.0061, -17.0119) (-19.9524, -16.9985) (-19.8989, -16.985) (-19.8455, -16.9712) (-19.7923, -16.9571) (-19.7392, -16.9428) (-19.6862, -16.9283) (-19.6334, -16.9135) (-19.5807, -16.8985) (-19.5282, -16.8832) (-19.4758, -16.8677) (-19.4236, -16.8519) (-19.3715, -16.8359) (-19.3196, -16.8196) (-19.2678, -16.8031) (-19.2162, -16.7863) (-19.1647, -16.7693) (-19.1134, -16.752) (-19.0623, -16.7344) (-19.0114, -16.7166) (-18.9606, -16.6985) (-18.91, -16.6801) (-18.8595, -16.6615) (-18.8093, -16.6426) (-18.7592, -16.6234) (-18.7093, -16.6039) (-18.6596, -16.5842) (-18.6102, -16.5641) (-18.5609, -16.5438) (-18.5118, -16.5232) (-18.4629, -16.5023) (-18.4142, -16.4811) (-18.3657, -16.4596) (-18.3174, -16.4378) (-18.2694, -16.4156) (-18.2217, -16.3931) (-18.1742, -16.3703) (-18.1269, -16.3471) (-18.0799, -16.3236) (-18.0331, -16.2998) (-17.9865, -16.2756) (-17.9402, -16.2512) (-17.8941, -16.2264) (-17.8484, -16.2012) (-17.8031, -16.1754) (-17.7582, -16.1491) (-17.7138, -16.1223) (-17.6697, -16.095) (-17.6259, -16.0673) (-17.5823, -16.0394) (-17.5389, -16.0113) (-17.4958, -15.9828) (-17.4534, -15.9536) (-17.4118, -15.9233) (-17.3795, -15.8978) (-17.356, -15.8779) (-17.3407, -15.8642) (-17.3331, -15.8573) knots -1 -1 -1 -1 -1 -1 -0.98571429 -0.97142857 -0.95714286 -0.94285714 -0.92857143 -0.91428571 -0.9 -0.88571429 -0.87142857 -0.85714286 -0.84285714 -0.82857143 -0.81428571 -0.8 -0.78571429 -0.77142857 -0.75714286 -0.74285714 -0.72857143 -0.71428571 -0.7 -0.68571429 -0.67142857 -0.65714286 -0.64285714 -0.62857143 -0.61428571 -0.6 -0.58571429 -0.57142857 -0.55714286 -0.54285714 -0.52857143 -0.51428571 -0.5 -0.48571429 -0.47142857 -0.45714286 -0.44285714 -0.42857143 -0.41428571 -0.4 -0.38571429 -0.37142857 -0.35714286 -0.34285714 -0.32857143 -0.31428571 -0.3 -0.28571429 -0.27142857 -0.25714286 -0.24285714 -0.22857143 -0.21428571 -0.2 -0.18571429 -0.17142857 -0.15714286 -0.14285714 -0.12857143 -0.11428571 -0.1 -0.08571429 -0.07142857 -0.05714286 -0.04285714 -0.02857143 -0.01428571 0 0 0 0 0 0
  line L21 (-17.3331, -15.8573) -> (-16.9653, -15.5213)
  arc A45 (-16.2666, -15.545) -> (-16.9653, -15.5213) centre (-16.6281, -15.8905) ccw
  arc A46 (-16.2666, -15.545) -> (-15.4311, -16.3747) centre (0, 0) ccw
  arc A47 (-15.4025, -17.0732) -> (-15.4311, -16.3747) centre (-15.774, -16.7386) ccw
  line L22 (-15.4025, -17.0732) -> (-15.7359, -17.4434)
  spline S20 degree 5 poles (-15.7359, -17.4434) (-15.7427, -17.451) (-15.7563, -17.4665) (-15.7761, -17.4901) (-15.8013, -17.5225) (-15.8313, -17.5643) (-15.8602, -17.607) (-15.8885, -17.6502) (-15.9163, -17.6938) (-15.9439, -17.7376) (-15.9712, -17.7816) (-15.9982, -17.8259) (-16.0247, -17.8705) (-16.0507, -17.9156) (-16.0762, -17.9611) (-16.1011, -18.007) (-16.1256, -18.0532) (-16.1497, -18.0997) (-16.1735, -18.1464) (-16.1969, -18.1934) (-16.2201, -18.2406) (-16.243, -18.288) (-16.2655, -18.3357) (-16.2877, -18.3836) (-16.3095, -18.4317) (-16.331, -18.4802) (-16.3521, -18.5288) (-16.373, -18.5776) (-16.3935, -18.6267) (-16.4138, -18.6759) (-16.4338, -18.7253) (-16.4535, -18.775) (-16.4729, -18.8248) (-16.492, -18.8748) (-16.5109, -18.925) (-16.5294, -18.9754) (-16.5477, -19.0259) (-16.5657, -19.0767) (-16.5834, -19.1276) (-16.6009, -19.1787) (-16.6181, -19.2299) (-16.6351, -19.2813) (-16.6517, -19.3329) (-16.6682, -19.3846) (-16.6843, -19.4365) (-16.7002, -19.4886) (-16.7159, -19.5407) (-16.7313, -19.5931) (-16.7464, -19.6456) (-16.7614, -19.6982) (-16.776, -19.751) (-16.7904, -19.8039) (-16.8046, -19.857) (-16.8185, -19.9102) (-16.8322, -19.9635) (-16.8456, -20.017) (-16.8588, -20.0706) (-16.8718, -20.1243) (-16.8845, -20.1782) (-16.897, -20.2322) (-16.9093, -20.2863) (-16.9213, -20.3406) (-16.9331, -20.3949) (-16.9446, -20.4494) (-16.956, -20.504) (-16.9671, -20.5587) (-16.9779, -20.6136) (-16.9886, -20.6686) (-16.999, -20.7236) (-17.0092, -20.7788) (-17.0191, -20.8341) (-17.0269, -20.8784) (-17.0326, -20.9117) (-17.0364, -20.934) (-17.0383, -20.9451) knots 0 0 0 0 0 0 0.01428571 0.02857143 0.04285714 0.05714286 0.07142857 0.08571429 0.1 0.11428571 0.12857143 0.14285714 0.15714286 0.17142857 0.18571429 0.2 0.21428571 0.22857143 0.24285714 0.25714286 0.27142857 0.28571429 0.3 0.31428571 0.32857143 0.34285714 0.35714286 0.37142857 0.38571429 0.4 0.41428571 0.42857143 0.44285714 0.45714286 0.47142857 0.48571429 0.5 0.51428571 0.52857143 0.54285714 0.55714286 0.57142857 0.58571429 0.6 0.61428571 0.62857143 0.64285714 0.65714286 0.67142857 0.68571429 0.7 0.71428571 0.72857143 0.74285714 0.75714286 0.77142857 0.78571429 0.8 0.81428571 0.82857143 0.84285714 0.85714286 0.87142857 0.88571429 0.9 0.91428571 0.92857143 0.94285714 0.95714286 0.97142857 0.98571429 1 1 1 1 1 1
  arc A48 (-17.0383, -20.9451) -> (-15.8978, -21.8234) centre (0, 0) ccw
  spline S21 degree 5 poles (-15.8978, -21.8234) (-15.8876, -21.8187) (-15.867, -21.8094) (-15.8363, -21.7953) (-15.7954, -21.7765) (-15.7445, -21.7527) (-15.6938, -21.7288) (-15.6432, -21.7046) (-15.5928, -21.6803) (-15.5425, -21.6558) (-15.4924, -21.6311) (-15.4425, -21.6062) (-15.3928, -21.5811) (-15.3433, -21.5558) (-15.2939, -21.5303) (-15.2447, -21.5047) (-15.1957, -21.4788) (-15.1468, -21.4527) (-15.0982, -21.4265) (-15.0498, -21.4) (-15.0015, -21.3734) (-14.9534, -21.3465) (-14.9055, -21.3195) (-14.8579, -21.2922) (-14.8104, -21.2647) (-14.7631, -21.2371) (-14.716, -21.2092) (-14.6691, -21.1812) (-14.6224, -21.1529) (-14.576, -21.1244) (-14.5297, -21.0958) (-14.4837, -21.0669) (-14.4379, -21.0378) (-14.3923, -21.0085) (-14.3469, -20.979) (-14.3018, -20.9493) (-14.2568, -20.9193) (-14.2121, -20.8892) (-14.1677, -20.8588) (-14.1235, -20.8282) (-14.0795, -20.7974) (-14.0358, -20.7664) (-13.9923, -20.7351) (-13.9491, -20.7036) (-13.9062, -20.6719) (-13.8635, -20.6399) (-13.821, -20.6078) (-13.7789, -20.5754) (-13.737, -20.5427) (-13.6954, -20.5098) (-13.6541, -20.4767) (-13.6131, -20.4433) (-13.5724, -20.4096) (-13.5321, -20.3757) (-13.4921, -20.3415) (-13.4524, -20.307) (-13.413, -20.2723) (-13.3738, -20.2374) (-13.335, -20.2022) (-13.2966, -20.1667) (-13.2586, -20.1309) (-13.2211, -20.0947) (-13.1842, -20.0581) (-13.1478, -20.021) (-13.1119, -19.9836) (-13.0763, -19.9459) (-13.041, -19.9081) (-13.006, -19.87) (-12.9714, -19.8317) (-12.9375, -19.7928) (-12.9048, -19.7531) (-12.8799, -19.7205) (-12.8621, -19.6953) (-12.8506, -19.6782) (-12.845, -19.6696) knots -1 -1 -1 -1 -1 -1 -0.98571429 -0.97142857 -0.95714286 -0.94285714 -0.92857143 -0.91428571 -0.9 -0.88571429 -0.87142857 -0.85714286 -0.84285714 -0.82857143 -0.81428571 -0.8 -0.78571429 -0.77142857 -0.75714286 -0.74285714 -0.72857143 -0.71428571 -0.7 -0.68571429 -0.67142857 -0.65714286 -0.64285714 -0.62857143 -0.61428571 -0.6 -0.58571429 -0.57142857 -0.55714286 -0.54285714 -0.52857143 -0.51428571 -0.5 -0.48571429 -0.47142857 -0.45714286 -0.44285714 -0.42857143 -0.41428571 -0.4 -0.38571429 -0.37142857 -0.35714286 -0.34285714 -0.32857143 -0.31428571 -0.3 -0.28571429 -0.27142857 -0.25714286 -0.24285714 -0.22857143 -0.21428571 -0.2 -0.18571429 -0.17142857 -0.15714286 -0.14285714 -0.12857143 -0.11428571 -0.1 -0.08571429 -0.07142857 -0.05714286 -0.04285714 -0.02857143 -0.01428571 0 0 0 0 0 0
  line L23 (-12.845, -19.6696) -> (-12.5723, -19.2528)
  arc A49 (-11.8897, -19.102) -> (-12.5723, -19.2528) centre (-12.1539, -19.5265) ccw
  arc A50 (-11.8897, -19.102) -> (-10.8741, -19.6978) centre (0, 0) ccw
  arc A51 (-10.6726, -20.3673) -> (-10.8741, -19.6978) centre (-11.1157, -20.1356) ccw
  line L24 (-10.6726, -20.3673) -> (-10.9035, -20.8087)
  spline S22 degree 5 poles (-10.9035, -20.8087) (-10.9083, -20.8178) (-10.9176, -20.8362) (-10.9308, -20.864) (-10.9472, -20.9016) (-10.9659, -20.9496) (-10.9833, -20.9981) (-10.9999, -21.047) (-11.016, -21.0962) (-11.0318, -21.1454) (-11.0474, -21.1949) (-11.0625, -21.2445) (-11.0771, -21.2943) (-11.091, -21.3444) (-11.1044, -21.3948) (-11.1171, -21.4454) (-11.1293, -21.4963) (-11.1411, -21.5473) (-11.1525, -21.5985) (-11.1636, -21.6498) (-11.1743, -21.7013) (-11.1846, -21.7529) (-11.1946, -21.8047) (-11.2041, -21.8566) (-11.2133, -21.9087) (-11.2221, -21.9609) (-11.2305, -22.0133) (-11.2385, -22.0658) (-11.2462, -22.1184) (-11.2536, -22.1711) (-11.2607, -22.224) (-11.2674, -22.2769) (-11.2738, -22.33) (-11.2799, -22.3832) (-11.2857, -22.4365) (-11.2911, -22.4899) (-11.2963, -22.5435) (-11.3011, -22.5971) (-11.3056, -22.6508) (-11.3098, -22.7046) (-11.3137, -22.7585) (-11.3174, -22.8125) (-11.3207, -22.8666) (-11.3237, -22.9208) (-11.3265, -22.9751) (-11.329, -23.0295) (-11.3311, -23.0839) (-11.333, -23.1384) (-11.3347, -23.1931) (-11.336, -23.2477) (-11.3371, -23.3025) (-11.3379, -23.3574) (-11.3384, -23.4123) (-11.3387, -23.4673) (-11.3387, -23.5223) (-11.3384, -23.5775) (-11.3378, -23.6327) (-11.337, -23.6879) (-11.336, -23.7433) (-11.3346, -23.7987) (-11.333, -23.8541) (-11.3312, -23.9097) (-11.3291, -23.9653) (-11.3267, -24.0209) (-11.3241, -24.0766) (-11.3213, -24.1324) (-11.3181, -24.1882) (-11.3148, -24.2441) (-11.3112, -24.3) (-11.3073, -24.356) (-11.3032, -24.4121) (-11.2997, -24.4569) (-11.297, -24.4906) (-11.2951, -24.5131) (-11.2942, -24.5243) knots 0 0 0 0 0 0 0.01428571 0.02857143 0.04285714 0.05714286 0.07142857 0.08571429 0.1 0.11428571 0.12857143 0.14285714 0.15714286 0.17142857 0.18571429 0.2 0.21428571 0.22857143 0.24285714 0.25714286 0.27142857 0.28571429 0.3 0.31428571 0.32857143 0.34285714 0.35714286 0.37142857 0.38571429 0.4 0.41428571 0.42857143 0.44285714 0.45714286 0.47142857 0.48571429 0.5 0.51428571 0.52857143 0.54285714 0.55714286 0.57142857 0.58571429 0.6 0.61428571 0.62857143 0.64285714 0.65714286 0.67142857 0.68571429 0.7 0.71428571 0.72857143 0.74285714 0.75714286 0.77142857 0.78571429 0.8 0.81428571 0.82857143 0.84285714 0.85714286 0.87142857 0.88571429 0.9 0.91428571 0.92857143 0.94285714 0.95714286 0.97142857 0.98571429 1 1 1 1 1 1
  arc A52 (-11.2942, -24.5243) -> (-9.9711, -25.0914) centre (0, 0) ccw
  spline S23 degree 5 poles (-9.9711, -25.0914) (-9.9623, -25.0843) (-9.9448, -25.0702) (-9.9185, -25.0489) (-9.8836, -25.0205) (-9.8402, -24.9848) (-9.797, -24.949) (-9.754, -24.913) (-9.7112, -24.877) (-9.6686, -24.8407) (-9.6263, -24.8043) (-9.5841, -24.7678) (-9.5422, -24.7311) (-9.5005, -24.6943) (-9.459, -24.6574) (-9.4178, -24.6203) (-9.3767, -24.583) (-9.3359, -24.5456) (-9.2953, -24.5081) (-9.255, -24.4704) (-9.2149, -24.4326) (-9.175, -24.3946) (-9.1353, -24.3565) (-9.0959, -24.3183) (-9.0567, -24.2799) (-9.0178, -24.2413) (-8.9791, -24.2026) (-8.9407, -24.1638) (-8.9025, -24.1248) (-8.8646, -24.0857) (-8.8269, -24.0464) (-8.7895, -24.007) (-8.7524, -23.9674) (-8.7155, -23.9277) (-8.6789, -23.8878) (-8.6426, -23.8478) (-8.6065, -23.8076) (-8.5707, -23.7673) (-8.5352, -23.7268) (-8.5, -23.6862) (-8.4651, -23.6454) (-8.4304, -23.6045) (-8.3961, -23.5634) (-8.3621, -23.5222) (-8.3284, -23.4808) (-8.295, -23.4392) (-8.2619, -23.3975) (-8.2291, -23.3556) (-8.1966, -23.3136) (-8.1645, -23.2714) (-8.1327, -23.229) (-8.1013, -23.1865) (-8.0703, -23.1437) (-8.0397, -23.1008) (-8.0095, -23.0577) (-7.9796, -23.0145) (-7.95, -22.9711) (-7.9209, -22.9275) (-7.892, -22.8838) (-7.8636, -22.8399) (-7.8357, -22.7957) (-7.8084, -22.7513) (-7.7818, -22.7067) (-7.7557, -22.6617) (-7.7302, -22.6166) (-7.7052, -22.5712) (-7.6804, -22.5258) (-7.656, -22.4802) (-7.632, -22.4345) (-7.6088, -22.3884) (-7.587, -22.3418) (-7.571, -22.304) (-7.56, -22.2752) (-7.5531, -22.2558) (-7.5498, -22.2461) knots -1 -1 -1 -1 -1 -1 -0.98571429 -0.97142857 -0.95714286 -0.94285714 -0.92857143 -0.91428571 -0.9 -0.88571429 -0.87142857 -0.85714286 -0.84285714 -0.82857143 -0.81428571 -0.8 -0.78571429 -0.77142857 -0.75714286 -0.74285714 -0.72857143 -0.71428571 -0.7 -0.68571429 -0.67142857 -0.65714286 -0.64285714 -0.62857143 -0.61428571 -0.6 -0.58571429 -0.57142857 -0.55714286 -0.54285714 -0.52857143 -0.51428571 -0.5 -0.48571429 -0.47142857 -0.45714286 -0.44285714 -0.42857143 -0.41428571 -0.4 -0.38571429 -0.37142857 -0.35714286 -0.34285714 -0.32857143 -0.31428571 -0.3 -0.28571429 -0.27142857 -0.25714286 -0.24285714 -0.22857143 -0.21428571 -0.2 -0.18571429 -0.17142857 -0.15714286 -0.14285714 -0.12857143 -0.11428571 -0.1 -0.08571429 -0.07142857 -0.05714286 -0.04285714 -0.02857143 -0.01428571 0 0 0 0 0 0
  line L25 (-7.5498, -22.2461) -> (-7.3894, -21.7745)
  arc A53 (-6.7657, -21.4587) -> (-7.3894, -21.7745) centre (-6.916, -21.9356) ccw
  arc A54 (-6.7657, -21.4587) -> (-5.6338, -21.7833) centre (0, 0) ccw
  arc A55 (-5.2722, -22.3816) -> (-5.6338, -21.7833) centre (-5.759, -22.2673) ccw
  line L26 (-5.2722, -22.3816) -> (-5.386, -22.8666)
  spline S24 degree 5 poles (-5.386, -22.8666) (-5.3884, -22.8766) (-5.3928, -22.8966) (-5.3988, -22.9269) (-5.4053, -22.9674) (-5.4114, -23.0185) (-5.4162, -23.0698) (-5.4201, -23.1213) (-5.4235, -23.1729) (-5.4266, -23.2246) (-5.4293, -23.2763) (-5.4317, -23.3282) (-5.4334, -23.3801) (-5.4344, -23.4321) (-5.4348, -23.4842) (-5.4346, -23.5364) (-5.4337, -23.5887) (-5.4325, -23.6411) (-5.4308, -23.6935) (-5.4288, -23.7459) (-5.4263, -23.7985) (-5.4235, -23.851) (-5.4203, -23.9036) (-5.4166, -23.9563) (-5.4125, -24.009) (-5.408, -24.0618) (-5.4032, -24.1146) (-5.3979, -24.1674) (-5.3923, -24.2203) (-5.3863, -24.2732) (-5.38, -24.3262) (-5.3734, -24.3792) (-5.3664, -24.4322) (-5.3591, -24.4852) (-5.3514, -24.5383) (-5.3434, -24.5914) (-5.335, -24.6445) (-5.3264, -24.6976) (-5.3174, -24.7508) (-5.3081, -24.8039) (-5.2985, -24.8571) (-5.2886, -24.9104) (-5.2783, -24.9636) (-5.2678, -25.0168) (-5.257, -25.0701) (-5.2458, -25.1233) (-5.2344, -25.1766) (-5.2227, -25.2299) (-5.2107, -25.2832) (-5.1984, -25.3365) (-5.1858, -25.3898) (-5.1729, -25.4432) (-5.1598, -25.4965) (-5.1464, -25.5498) (-5.1327, -25.6031) (-5.1187, -25.6565) (-5.1044, -25.7098) (-5.0899, -25.7631) (-5.0751, -25.8165) (-5.06, -25.8698) (-5.0447, -25.9231) (-5.0291, -25.9765) (-5.0132, -26.0298) (-4.9971, -26.0831) (-4.9807, -26.1364) (-4.9641, -26.1897) (-4.9472, -26.243) (-4.93, -26.2963) (-4.9126, -26.3496) (-4.895, -26.4028) (-4.8771, -26.4561) (-4.8625, -26.4987) (-4.8515, -26.5306) (-4.8441, -26.5519) (-4.8404, -26.5626) knots 0 0 0 0 0 0 0.01428571 0.02857143 0.04285714 0.05714286 0.07142857 0.08571429 0.1 0.11428571 0.12857143 0.14285714 0.15714286 0.17142857 0.18571429 0.2 0.21428571 0.22857143 0.24285714 0.25714286 0.27142857 0.28571429 0.3 0.31428571 0.32857143 0.34285714 0.35714286 0.37142857 0.38571429 0.4 0.41428571 0.42857143 0.44285714 0.45714286 0.47142857 0.48571429 0.5 0.51428571 0.52857143 0.54285714 0.55714286 0.57142857 0.58571429 0.6 0.61428571 0.62857143 0.64285714 0.65714286 0.67142857 0.68571429 0.7 0.71428571 0.72857143 0.74285714 0.75714286 0.77142857 0.78571429 0.8 0.81428571 0.82857143 0.84285714 0.85714286 0.87142857 0.88571429 0.9 0.91428571 0.92857143 0.94285714 0.95714286 0.97142857 0.98571429 1 1 1 1 1 1
  arc A56 (-4.8404, -26.5626) -> (-3.4179, -26.7828) centre (0, 0) ccw
  spline S25 degree 5 poles (-3.4179, -26.7828) (-3.4111, -26.7738) (-3.3976, -26.7557) (-3.3775, -26.7286) (-3.3508, -26.6924) (-3.3176, -26.647) (-3.2846, -26.6016) (-3.2519, -26.5561) (-3.2195, -26.5105) (-3.1872, -26.4648) (-3.1553, -26.419) (-3.1235, -26.3731) (-3.092, -26.3272) (-3.0608, -26.2812) (-3.0298, -26.2351) (-2.9991, -26.1889) (-2.9686, -26.1426) (-2.9384, -26.0962) (-2.9084, -26.0498) (-2.8787, -26.0032) (-2.8492, -25.9566) (-2.82, -25.9099) (-2.7911, -25.8632) (-2.7624, -25.8163) (-2.7341, -25.7694) (-2.7059, -25.7224) (-2.6781, -25.6753) (-2.6505, -25.6281) (-2.6233, -25.5809) (-2.5962, -25.5335) (-2.5695, -25.4861) (-2.5431, -25.4386) (-2.517, -25.3911) (-2.4911, -25.3434) (-2.4656, -25.2957) (-2.4403, -25.2479) (-2.4154, -25.2) (-2.3908, -25.1521) (-2.3664, -25.104) (-2.3424, -25.0559) (-2.3187, -25.0077) (-2.2954, -24.9595) (-2.2723, -24.9112) (-2.2496, -24.8627) (-2.2273, -24.8143) (-2.2053, -24.7657) (-2.1836, -24.7171) (-2.1623, -24.6683) (-2.1413, -24.6196) (-2.1207, -24.5707) (-2.1004, -24.5218) (-2.0806, -24.4727) (-2.0612, -24.4236) (-2.0422, -24.3745) (-2.0236, -24.3252) (-2.0054, -24.2759) (-1.9876, -24.2265) (-1.9702, -24.177) (-1.9531, -24.1275) (-1.9365, -24.0779) (-1.9205, -24.0282) (-1.9051, -23.9784) (-1.8904, -23.9285) (-1.8763, -23.8785) (-1.8629, -23.8285) (-1.8499, -23.7783) (-1.8372, -23.7281) (-1.8248, -23.6779) (-1.813, -23.6277) (-1.802, -23.5773) (-1.7924, -23.5267) (-1.7863, -23.4861) (-1.7829, -23.4555) (-1.781, -23.435) (-1.7802, -23.4248) knots -1 -1 -1 -1 -1 -1 -0.98571429 -0.97142857 -0.95714286 -0.94285714 -0.92857143 -0.91428571 -0.9 -0.88571429 -0.87142857 -0.85714286 -0.84285714 -0.82857143 -0.81428571 -0.8 -0.78571429 -0.77142857 -0.75714286 -0.74285714 -0.72857143 -0.71428571 -0.7 -0.68571429 -0.67142857 -0.65714286 -0.64285714 -0.62857143 -0.61428571 -0.6 -0.58571429 -0.57142857 -0.55714286 -0.54285714 -0.52857143 -0.51428571 -0.5 -0.48571429 -0.47142857 -0.45714286 -0.44285714 -0.42857143 -0.41428571 -0.4 -0.38571429 -0.37142857 -0.35714286 -0.34285714 -0.32857143 -0.31428571 -0.3 -0.28571429 -0.27142857 -0.25714286 -0.24285714 -0.22857143 -0.21428571 -0.2 -0.18571429 -0.17142857 -0.15714286 -0.14285714 -0.12857143 -0.11428571 -0.1 -0.08571429 -0.07142857 -0.05714286 -0.04285714 -0.02857143 -0.01428571 0 0 0 0 0 0
  line L27 (-1.7802, -23.4248) -> (-1.7421, -22.9281)
  arc A57 (-1.2165, -22.4671) -> (-1.7421, -22.9281) centre (-1.2436, -22.9664) ccw
  arc A58 (-1.2165, -22.4671) -> (-0.0395, -22.5) centre (0, 0) ccw
  arc A59 (0.4595, -22.9896) -> (-0.0395, -22.5) centre (-0.0404, -23) ccw
  line L28 (0.4595, -22.9896) -> (0.4699, -23.4876)